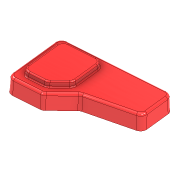
# Autodesk Inventor part: Plastic Cover
Saved by Autodesk Inventor 2020.1 (Build 241239000, 239)
## iProperties
Created: 2019-09-07
Part Number: Plastic Cover
Material: Generic
Document SubType Name: Modeling
Designer: thom_tremblay
Density: 1 g/cm^3
Appearance: Light Red
Author: thom_tremblay
Autodesk Inventor part; units mm, degrees
ref_plane "YZ Plane" through (0, 0, 0) normal (1, 0, 0) x (0, 1, 0)
ref_plane "XZ Plane" through (0, 0, 0) normal (0, 1, 0) x (-1, 0, 0)
ref_plane "XY Plane" through (0, 0, 0) normal (0, 0, 1) x (1, 0, 0)
sketch "Sketch1" plane through (0, 0, 0) normal (0, 0, 1) x (1, 0, 0)
  line L0 (0, 0) -> (0, 208.28)
  line L1 (0, 208.28) -> (-114.3, 208.28)
  line L2 (-114.3, 208.28) -> (-184.237, 149.5959)
  line L3 (-184.237, 149.5959) -> (-355.6, 119.38)
  line L4 (-355.6, 119.38) -> (-355.6, 0)
  line L5 (-355.6, 0) -> (0, 0)
  dimension "d0" = 208.28
  dimension "d1" = 355.6
  dimension "d2" = 100
  dimension "d3" = 140
  dimension "d4" = 114.3
  dimension "d5" = 119.38
  constraints: 12 end point, 2 perpendicular, 1 parallel, 1 vertical
  measures "d0" distance of L0.start L0.end
  measures "d1" distance of L4.end L0.start
  measures "d2" angle of L3 L4
  measures "d3" angle of L1 L2
  measures "d4" distance of L0.end L1.end
  measures "d5" distance of L3.end L4.end
extrude "Extrusion1" add sketch "Sketch1" along normal blind 50.8 draft -2
sketch "Sketch2" plane through (0, 0, 50.8) normal (0, 0, 1) x (1, 0, 0)
  point P0 (0, 0)
sketch "Sketch3" plane through (0, 0, 50.8) normal (0, 0, 1) x (1, 0, 0)
  line L0 (-113.6543, 206.506) -> (-1.774, 206.506) construction
  line L1 (-183.4608, 147.9314) -> (-113.6543, 206.506) construction
  line L2 (-353.826, 117.8915) -> (-183.4608, 147.9314) construction
  line L3 (-353.826, 1.774) -> (-353.826, 117.8915) construction
  line L4 (-1.774, 1.774) -> (-353.826, 1.774) construction
  line L5 (-1.774, 206.506) -> (-1.774, 1.774) construction
  line L6 (-154.174, 27.174) -> (-27.174, 27.174)
  line L7 (-27.174, 27.174) -> (-27.174, 181.106)
  line L8 (-27.174, 181.106) -> (-104.4095, 181.106)
  line L9 (-104.4095, 181.106) -> (-154.174, 139.3487)
  line L10 (-154.174, 139.3487) -> (-154.174, 27.174)
  line L11 (-27.174, 27.174) -> (-27.174, 1.774) construction
  line L12 (0, 1.774) -> (-353.826, 1.774) projected
  line L13 (-27.174, 181.106) -> (-1.774, 181.106) construction
  line L14 (-1.774, 206.506) -> (-1.774, 0) projected
  line L15 (-27.174, 181.106) -> (-27.174, 206.506) construction
  line L16 (-154.174, 139.3487) -> (-170.5008, 158.8062) construction
  line L17 (-183.4608, 147.9314) -> (-113.6543, 206.506) construction
  point P0 (0, 0)
  dimension "d8" = 25.4
  dimension "d9" = 127
  constraints: 18 end point, 5 perpendicular, 3 equal length, 3 point on line, 2 parallel, 1 horizontal, 4 other
  measures "d8" distance between parallel lines of L1 L9
  measures "d9" distance of L6.start L6.end
extrude "Extrusion2" add sketch "Sketch3" along normal blind 17.78 draft -2
fillet "Fillet1" radius 20.32 6 edges at (-354.713, 118.6357, 25.4) (-354.713, 0.887, 25.4) (-183.8489, 148.7637, 25.4) (-113.9772, 207.393, 25.4) (-0.887, 207.393, 25.4) (-0.887, 0.887, 25.4)
fillet "Fillet1" radius 20.32 5 edges at (-27.4844, 180.7956, 59.69) (-27.4844, 27.4844, 59.69) (-104.2965, 180.7956, 59.69) (-153.8635, 139.2039, 59.69) (-153.8635, 27.4844, 59.69)
fillet "Fillet1" radius 3.81 5 edges at (-154.174, 83.2613, 50.8) (-129.2917, 160.2273, 50.8) (-65.7917, 181.106, 50.8) (-27.174, 104.14, 50.8) (-90.674, 27.174, 50.8)
fillet "Fillet1" radius 7.62 6 edges at (-57.7142, 206.506, 50.8) (-148.5576, 177.2187, 50.8) (-268.6434, 132.9115, 50.8) (-353.826, 59.8327, 50.8) (-177.8, 1.774, 50.8) (-1.774, 104.14, 50.8)
fillet "Fillet1" radius 4.572 5 edges at (-90.674, 27.7949, 68.58) (-27.7949, 104.14, 68.58) (-65.9892, 180.4851, 68.58) (-128.8683, 159.7721, 68.58) (-153.5531, 83.427, 68.58)
shell "Shell1" thickness 3.81 removed faces 1 at (-181.7319, 49.5503, 0)
sketch "Sketch4" plane through (0, 0, 68.58) normal (0, 0, 1) x (1, 0, 0)
  line L0 (-50.8, 46.99) -> (-127, 46.99)
  line L1 (-127, 46.99) -> (-127, 87.63)
  line L2 (-127, 87.63) -> (-50.8, 87.63)
  line L3 (-50.8, 87.63) -> (-50.8, 46.99)
  line L4 (-50.8, 87.63) -> (-81.28, 87.63)
  line L5 (-81.28, 87.63) -> (-81.28, 118.11)
  line L6 (-81.28, 118.11) -> (-50.8, 118.11)
  line L7 (-50.8, 118.11) -> (-50.8, 87.63)
  point P0 (0, 0)
  dimension "d18" = 46.99
  dimension "d19" = 50.8
  dimension "d20" = 76.2
  dimension "d21" = 71.12
  dimension "d22" = 30.48
  dimension "d23" = 40.64
  constraints: 16 end point, 4 parallel, 2 horizontal, 2 perpendicular
  measures "d18" distance from line of L0 point (0, 0)
  measures "d19" distance from line of L3 point (0, 0)
  measures "d20" distance of L0.start L0.end
  measures "d21" distance between parallel lines of L6 L0
  measures "d22" distance of L5.end L6.end
  measures "d23" distance of L2.end L0.start
body "Solid1"
